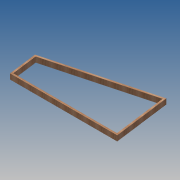
# Autodesk Inventor part: panelBflat
Saved by Autodesk Inventor 2014 SP1 (Build 180222100, 222)
## iProperties
Created: 2015-02-12
Part Number: panelBflat
Material: Wood (Birch)
Document SubType Name: Modeling
Designer: Dave
Density: 0.55 g/cm^3
Appearance: Birch - Natural Polished
Mass: 14992.5 g
Surface Area: 19129.1 cm^2
Volume: 27259 cm^3
Author: Dave
Autodesk Inventor part; units mm, degrees
ref_plane "YZ Plane" through (0, 0, 0) normal (1, 0, 0) x (0, 1, 0)
ref_plane "XZ Plane" through (0, 0, 0) normal (0, 1, 0) x (-1, 0, 0)
ref_plane "XY Plane" through (0, 0, 0) normal (0, 0, 1) x (1, 0, 0)
sketch "Sketch1" plane through (0, 0, 0) normal (0, 1, 0) x (-1, 0, 0)
  line L0 (0, 0) -> (-4300, 0) construction
  line L1 (0, 0) -> (-4153.4811, -1112.9219) construction
  line L2 (0, 0) -> (4300, 0) construction
  line L3 (-4300, 0) -> (-4200, 0) construction
  line L4 (-2006.9086, 50) -> (-4306.5826, 50)
  line L5 (-4153.4811, -1112.9219) -> (-3780.7254, -1112.9219) construction
  line L6 (-1925.5839, -567.7225) -> (-4146.8984, -1162.9219)
  line L7 (-4146.8984, -1162.9219) -> (-4306.5826, 50)
  line L8 (-1925.5839, -567.7225) -> (-2006.9086, 50)
  line L9 (-4263.2519, 12) -> (-2040.2337, 12)
  line L10 (-2040.2337, 12) -> (-1967.6086, -539.6424)
  line L11 (-1967.6086, -539.6424) -> (-4114.8793, -1115.0019)
  line L12 (-4114.8793, -1115.0019) -> (-4263.2519, 12)
  dimension "d0" = 4300
  dimension "d1" = 4300
  dimension "d2" = 165
  dimension "d5" = 50
  dimension "d7" = 50
  dimension "d8" = 2280
  dimension "d11" = 38
  constraints: 26 end point, 4 horizontal, 2 parallel, 1 equal length, 3 other
  measures "d0" distance of L0.start L0.end
  measures "d1" distance of L0.start L1.end
  measures "d2" angle of L1 L2
  measures "d5" distance between parallel lines of L4 L0
  measures "d7" distance between parallel lines of L6 L1
  measures "d8" distance between parallel lines of L7 L8
  measures "d11" distance between parallel lines of L9 L4
extrude "Extrusion2" add sketch "Sketch1" along normal blind 114
body "Solid2"
